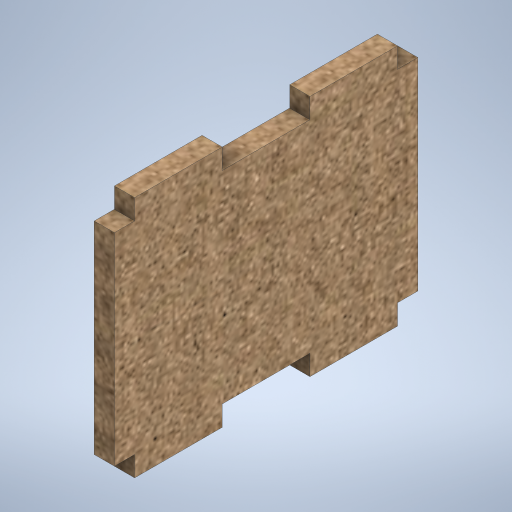
# Autodesk Inventor part: Case_Wall2
Saved by Autodesk Inventor 2024 (Build 280153000, 153)
## iProperties
Created: 2023-11-23
Part Number: Case_Wall2
Material: MDF Tablero de fibras de densidad media
Document SubType Name: Modeling
Designer: marco
Density: 0.8 g/cm^3
Appearance: Cartón - Ondulado
Author: marco
Autodesk Inventor part; units mm, degrees
ref_plane "YZ Plane" through (0, 0, 0) normal (1, 0, 0) x (0, 1, 0)
ref_plane "XZ Plane" through (0, 0, 0) normal (0, 1, 0) x (-1, 0, 0)
ref_plane "XY Plane" through (0, 0, 0) normal (0, 0, 1) x (1, 0, 0)
sketch "Boceto1" plane through (0, 0, 0) normal (1, 0, 0) x (0, 1, 0)
  line L0 (15, -6.5) -> (15, 6.5)
  line L1 (18, -6.5) -> (15, -6.5)
  line L2 (18, -19.5) -> (18, -6.5)
  line L3 (15, -19.5) -> (18, -19.5)
  line L4 (15, -22.5) -> (15, -19.5)
  line L5 (-15, -22.5) -> (15, -22.5)
  line L6 (-15, -19.5) -> (-15, -22.5)
  line L7 (-18, -19.5) -> (-15, -19.5)
  line L8 (-18, -6.5) -> (-18, -19.5)
  line L9 (-15, -6.5) -> (-18, -6.5)
  line L10 (-15, 6.5) -> (-15, -6.5)
  line L11 (-18, 6.5) -> (-15, 6.5)
  line L12 (-18, 19.5) -> (-18, 6.5)
  line L13 (-15, 19.5) -> (-18, 19.5)
  line L14 (-15, 22.5) -> (-15, 19.5)
  line L15 (15, 22.5) -> (-15, 22.5)
  line L16 (15, 19.5) -> (15, 22.5)
  line L17 (18, 19.5) -> (15, 19.5)
  line L18 (18, 6.5) -> (18, 19.5)
  line L19 (15, 6.5) -> (18, 6.5)
  point P0 (0, 0)
  constraints: 40 end point
extrude "Extrusión1" add sketch "Boceto1" along normal blind 3
